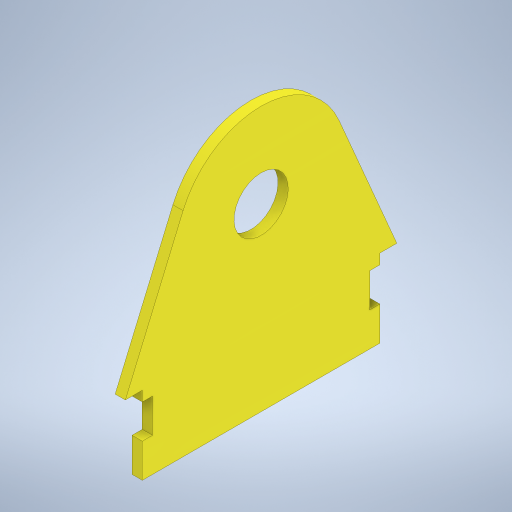
# Autodesk Inventor part: baseSoporte
Saved by Autodesk Inventor 2024.3 (Build 283343000, 343)
## iProperties
Created: 2024-05-14
Part Number: baseSoporte
Material: PMMA Plastic
Document SubType Name: Modeling
Designer: USUARIO
Density: 1.188 g/cm^3
Appearance: Canary
Mass: 15.1746 g
Surface Area: 94.6312 cm^2
Volume: 12.7732 cm^3
Author: USUARIO
Autodesk Inventor part; units mm, degrees
ref_plane "YZ Plane" through (0, 0, 0) normal (1, 0, 0) x (0, 1, 0)
ref_plane "XZ Plane" through (0, 0, 0) normal (0, 1, 0) x (-1, 0, 0)
ref_plane "XY Plane" through (0, 0, 0) normal (0, 0, 1) x (1, 0, 0)
sketch "Sketch1" plane through (0, 0, 0) normal (1, 0, 0) x (0, 1, 0)
  circle A0 centre (0, 0) radius 8
  arc A1 (-25, 0) -> (9.8205, -22.9904) centre (0, 0) ccw construction
  line L0 (-30, 0) -> (-30, -35) construction
  line L1 (-30, -40) -> (9.8205, -22.9904)
  line L2 (-30, 40) -> (9.8205, 22.9904)
  line L3 (-30, 0) -> (-33, 0) construction
  line L4 (-33, 0) -> (-33, -32) construction
  line L5 (-33, -35) -> (-30, -35)
  line L6 (-33, 0) -> (-33, 32) construction
  line L7 (-43, 35) -> (-46, 35)
  line L8 (-46, 35) -> (-46, -35) construction
  line L9 (-30, -35) -> (-30, -40)
  arc A2 (9.8205, 22.9904) -> (-25, 0) centre (0, 0) ccw construction
  arc A3 (9.8205, -22.9904) -> (9.8205, 22.9904) centre (0, 0) ccw
  line L10 (-30, 40) -> (-30, 35)
  line L11 (-30, 35) -> (-33, 35)
  line L12 (-43, 32) -> (-43, 35)
  line L13 (-33, -35) -> (-33, -32)
  line L14 (-33, -32) -> (-43, -32)
  line L15 (-43, -32) -> (-43, -35)
  line L16 (-43, -35) -> (-46, -35)
  line L17 (-33, 35) -> (-33, 32)
  line L18 (-33, 32) -> (-43, 32)
  line L19 (-46, 35) -> (-53, 35)
  line L20 (-53, 35) -> (-53, -35)
  line L21 (-53, -35) -> (-46, -35)
  dimension "d0" = 16
  dimension "d1" = 50
  dimension "d2" = 30
  dimension "d4" = 40
  dimension "d5" = 40
  dimension "d8" = 3
  dimension "d15" = 70
  dimension "d16" = 35
  dimension "d24" = 5
  dimension "d25" = 39.8205
  dimension "d27" = 3
  dimension "d28" = 3
  dimension "d29" = 3
  dimension "d30" = 10
  dimension "d31" = 3
  dimension "d32" = 3
  dimension "d33" = 3
  dimension "d34" = 10
  dimension "d35" = 7
  dimension "d36" = 70
  dimension "d37" = 7
  constraints: 44 end point, 10 perpendicular, 6 point on circle, 4 centre point, 4 tangent, 4 vertical, 3 horizontal, 2 coincident, 2 point on line, 1 collinear
  measures "d0" diameter of A0
  measures "d1" diameter of A1
  measures "d2" distance of A1.centre L0.start
  measures "d4" distance of L0.start L1.start
  measures "d5" distance of L0.start L2.start
  measures "d8" distance of L0.start L3.end
  measures "d15" distance of L8.end L7.end
  measures "d16" distance between parallel lines of L5 L3
  measures "d24" distance of L2.start L10.end
  measures "d25" horizontal distance of L2.end L2.start
  measures "d27" distance of L7.start L7.end
  measures "d28" distance of L5.start L0.end
  measures "d29" distance of L5.start L4.end
  measures "d30" distance of L4.end L14.end
  measures "d31" distance of L14.end L15.end
  measures "d32" distance of L15.end L8.end
  measures "d33" distance of L11.end L6.end
  measures "d34" distance of L6.end L12.start
  measures "d35" distance of L7.end L19.end
  measures "d36" distance of L19.end L20.end
  measures "d37" distance of L20.end L8.end
extrude "Extrusion1" add sketch "Sketch1" along normal blind 3
body "Solid1"
